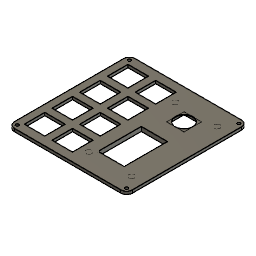
Top Plate (Autodesk Fusion 360 design; units mm, degrees)
part number: 2026-05-17-10-10-12-602
Autodesk Fusion 360 part; units mm, degrees
(part 1 of 3)
box "BoxPrimitive1" add length 100 width 50 height 2.5 placed x (0, 0, 1) y (1, 0, 0) z (0, 1, 0) at (0, 0, 0)
sketch "Sketch2" plane through (0, 2.5, 0) normal (0, 1, 0) x (-1, 0, 0)
  line L0 (0, 100) -> (-50, 100)
  line L1 (-50, 100) -> (-50, 0)
  line L2 (-50, 0) -> (0, 0)
  line L3 (0, 0) -> (0, 100)
  line L4 (-5, 95) -> (-19, 95)
  line L5 (-19, 95) -> (-19, 81)
  line L6 (-19, 81) -> (-5, 81)
  line L7 (-5, 81) -> (-5, 95)
  line L8 (-5, 95) -> (-19, 81) construction
  line L9 (-19, 95) -> (-5, 81) construction
  line L10 (-24.05, 95) -> (-38.05, 95)
  line L11 (-38.05, 95) -> (-38.05, 81)
  line L12 (-38.05, 81) -> (-24.05, 81)
  line L13 (-24.05, 81) -> (-24.05, 95)
  line L14 (-24.05, 95) -> (-38.05, 81) construction
  line L15 (-38.05, 95) -> (-24.05, 81) construction
  line L16 (-12, 88) -> (-31.05, 88)
  line L17 (-31.05, 88) -> (-31.05, 68.95)
  line L18 (-24.05, 75.95) -> (-38.05, 75.95)
  line L19 (-38.05, 75.95) -> (-38.05, 61.95)
  line L20 (-38.05, 61.95) -> (-24.05, 61.95)
  line L21 (-24.05, 61.95) -> (-24.05, 75.95)
  line L22 (-24.05, 75.95) -> (-38.05, 61.95) construction
  line L23 (-38.05, 75.95) -> (-24.05, 61.95) construction
  line L24 (-31.05, 68.95) -> (-31.05, 49.9)
  line L25 (-31.05, 49.9) -> (-12, 49.9)
  line L26 (-12, 49.9) -> (-12, 30.85)
  line L27 (-12, 30.85) -> (-31.05, 30.85)
  line L28 (-31.05, 30.85) -> (-31.05, 11.8)
  line L29 (-31.05, 11.8) -> (-12, 11.8)
  line L30 (-12, 49.9) -> (-12, 68.95)
  line L31 (-5, 61.95) -> (-19, 61.95)
  line L32 (-19, 61.95) -> (-19, 75.95)
  line L33 (-19, 75.95) -> (-5, 75.95)
  line L34 (-5, 75.95) -> (-5, 61.95)
  line L35 (-5, 61.95) -> (-19, 75.95) construction
  line L36 (-19, 61.95) -> (-5, 75.95) construction
  line L37 (-5, 56.9) -> (-19, 56.9)
  line L38 (-19, 56.9) -> (-19, 42.9)
  line L39 (-19, 42.9) -> (-5, 42.9)
  line L40 (-5, 42.9) -> (-5, 56.9)
  line L41 (-5, 56.9) -> (-19, 42.9) construction
  line L42 (-19, 56.9) -> (-5, 42.9) construction
  line L43 (-24.05, 42.9) -> (-38.05, 42.9)
  line L44 (-38.05, 42.9) -> (-38.05, 56.9)
  line L45 (-38.05, 56.9) -> (-24.05, 56.9)
  line L46 (-24.05, 56.9) -> (-24.05, 42.9)
  line L47 (-24.05, 42.9) -> (-38.05, 56.9) construction
  line L48 (-38.05, 42.9) -> (-24.05, 56.9) construction
  line L49 (-24.05, 23.85) -> (-38.05, 23.85)
  line L50 (-38.05, 23.85) -> (-38.05, 37.85)
  line L51 (-38.05, 37.85) -> (-24.05, 37.85)
  line L52 (-24.05, 37.85) -> (-24.05, 23.85)
  line L53 (-24.05, 23.85) -> (-38.05, 37.85) construction
  line L54 (-38.05, 23.85) -> (-24.05, 37.85) construction
  line L55 (-5, 23.85) -> (-19, 23.85)
  line L56 (-19, 23.85) -> (-19, 37.85)
  line L57 (-19, 37.85) -> (-5, 37.85)
  line L58 (-5, 37.85) -> (-5, 23.85)
  line L59 (-5, 23.85) -> (-19, 37.85) construction
  line L60 (-19, 23.85) -> (-5, 37.85) construction
  point P0 (-12, 88)
  point P1 (-31.05, 88)
  point P2 (-31.05, 68.95)
  point P3 (-12, 68.95)
  point P4 (-12, 49.9)
  point P5 (-31.05, 49.9)
  point P6 (-31.05, 30.85)
  point P7 (-12, 30.85)
  dimension "d8" = 14
  dimension "d9" = 14
  dimension "d10" = 14
  dimension "d11" = 14
  dimension "d12" = 19.05
  dimension "d13" = 19.05
  dimension "d14" = 14
  dimension "d15" = 14
  dimension "d16" = 19.05
  dimension "d17" = 19.05
  dimension "d18" = 19.05
  dimension "d19" = 19.05
  dimension "d20" = 19.05
  dimension "d21" = 19.05
  dimension "d22" = 19.05
  dimension "d23" = 14
  dimension "d24" = 14
  dimension "d25" = 14
  dimension "d26" = 14
  dimension "d27" = 14
  dimension "d28" = 14
  dimension "d29" = 14
  dimension "d30" = 14
  dimension "d31" = 14
  dimension "d32" = 14
  constraint horizontal L4
  constraint perpendicular L4 L5
  constraint parallel L4 L6
  constraint parallel L5 L7
  constraint coincident L8 P0
  constraint coincident L9 P0
  constraint horizontal L10
  constraint perpendicular L10 L11
  constraint parallel L10 L12
  constraint parallel L11 L13
  constraint coincident L14 P1
  constraint coincident L15 P1
  constraint coincident P0 L16.start
  constraint parallel L6 L16
  constraint coincident P1 L16.end
  constraint perpendicular L12 L17
  constraint horizontal L18
  constraint perpendicular L18 L19
  constraint parallel L18 L20
  constraint parallel L19 L21
  constraint coincident L22 P2
  constraint coincident L23 P2
  constraint coincident P2 L17.end
  constraint perpendicular L20 L24
  constraint perpendicular L24 L25
  constraint perpendicular L25 L26
  constraint perpendicular L26 L27
  constraint perpendicular L27 L28
  constraint perpendicular L28 L29
  constraint perpendicular L25 L30
  constraint horizontal L31
  constraint perpendicular L31 L32
  constraint parallel L31 L33
  constraint parallel L32 L34
  constraint coincident L35 P3
  constraint coincident L36 P3
  constraint coincident P3 L30.end
  constraint horizontal L37
  constraint perpendicular L37 L38
  constraint parallel L37 L39
  constraint parallel L38 L40
  constraint coincident L41 P4
  constraint coincident L42 P4
  constraint coincident P4 L25.end
  constraint horizontal L43
  constraint perpendicular L43 L44
  constraint parallel L43 L45
  constraint parallel L44 L46
  constraint coincident L47 P5
  constraint coincident L48 P5
  constraint coincident P5 L24.end
  constraint horizontal L49
  constraint perpendicular L49 L50
  constraint parallel L49 L51
  constraint parallel L50 L52
  constraint coincident L53 P6
  constraint coincident L54 P6
  constraint coincident P6 L27.end
  constraint horizontal L55
  constraint perpendicular L55 L56
  constraint parallel L55 L57
  constraint parallel L56 L58
  constraint coincident L59 P7
  constraint coincident L60 P7
  constraint coincident P7 L26.end
  measures "d8" distance of L5.end L6.end
  measures "d9" distance of L4.end L5.end
  measures "d10" distance of L11.end L12.end
  measures "d11" distance of L10.end L11.end
  measures "d12" distance of P0 P1
  measures "d13" distance of P1 P2
  measures "d14" distance of L19.end L20.end
  measures "d15" distance of L18.end L19.end
  measures "d16" distance of P2 P5
  measures "d17" distance of P5 P4
  measures "d18" distance of P4 P7
  measures "d19" distance of P7 P6
  measures "d20" distance of P6 L28.end
  measures "d21" distance of L28.end L29.end
  measures "d22" distance of P4 P3
  measures "d23" distance of L32.end L33.end
  measures "d24" distance of L31.end L32.end
  measures "d25" distance of L38.end L39.end
  measures "d26" distance of L37.end L38.end
  measures "d27" distance of L44.end L45.end
  measures "d28" distance of L43.end L44.end
  measures "d29" distance of L50.end L51.end
  measures "d30" distance of L49.end L50.end
  measures "d31" distance of L56.end L57.end
  measures "d32" distance of L55.end L56.end
extrude "Extrude1" cut sketch "Sketch2" against normal blind 10 contours L4 L5 L6 L7 | L10 L11 L12 L13 L16 L17 | L12 L13 L16 L17 | L17 L18 L20 L21 L24 | L17 L18 L19 L20 L24 | L24 L25 L45 L46 | L24 L25 L43 L44 L45 L46 | L25 L30 L37 L38 | L25 L26 L38 L39 | L26 L30 L37 L39 L40 | L26 L27 L55 L56 L57 L58 | L26 L27 L56 L57 | L27 L28 L49 L52 | L27 L28 L49 L50 L51 L52 | L31 L32 L33 L34
sketch "Sketch3" plane through (0, 2.5, 0) normal (0, 1, 0) x (-1, 0, 0)
  line L0 (0, 100) -> (-50, 100)
  line L1 (-50, 100) -> (-50, 0)
  line L2 (-50, 0) -> (0, 0)
  line L3 (0, 0) -> (0, 100)
  line L4 (-38.05, 95) -> (-24.05, 95)
  line L5 (-24.05, 95) -> (-24.05, 81)
  line L6 (-24.05, 81) -> (-38.05, 81)
  line L7 (-38.05, 81) -> (-38.05, 95)
  line L8 (-19, 61.95) -> (-19, 75.95)
  line L9 (-19, 75.95) -> (-5, 75.95)
  line L10 (-5, 75.95) -> (-5, 61.95)
  line L11 (-5, 61.95) -> (-19, 61.95)
  line L12 (-38.05, 23.85) -> (-38.05, 37.85)
  line L13 (-38.05, 37.85) -> (-24.05, 37.85)
  line L14 (-24.05, 37.85) -> (-24.05, 23.85)
  line L15 (-24.05, 23.85) -> (-38.05, 23.85)
  line L16 (-19, 95) -> (-5, 95)
  line L17 (-5, 95) -> (-5, 81)
  line L18 (-5, 81) -> (-19, 81)
  line L19 (-19, 81) -> (-19, 95)
  line L20 (-38.05, 75.95) -> (-24.05, 75.95)
  line L21 (-24.05, 75.95) -> (-24.05, 61.95)
  line L22 (-24.05, 61.95) -> (-38.05, 61.95)
  line L23 (-38.05, 61.95) -> (-38.05, 75.95)
  line L24 (-19, 56.9) -> (-5, 56.9)
  line L25 (-5, 56.9) -> (-5, 42.9)
  line L26 (-5, 42.9) -> (-19, 42.9)
  line L27 (-19, 42.9) -> (-19, 56.9)
  line L28 (-19, 23.85) -> (-19, 37.85)
  line L29 (-19, 37.85) -> (-5, 37.85)
  line L30 (-5, 37.85) -> (-5, 23.85)
  line L31 (-5, 23.85) -> (-19, 23.85)
  line L32 (-38.05, 42.9) -> (-38.05, 56.9)
  line L33 (-38.05, 56.9) -> (-24.05, 56.9)
  line L34 (-24.05, 56.9) -> (-24.05, 42.9)
  line L35 (-24.05, 42.9) -> (-38.05, 42.9)
  line L36 (-38.05, 23.85) -> (-38.05, 18.85)
  line L37 (-38.05, 18.85) -> (-43.05, 18.85)
  line L38 (-43.05, 18.85) -> (0, 18.85)
  line L39 (0, 18.85) -> (0, 100)
  line L40 (0, 100) -> (-43.05, 100)
  line L41 (-43.05, 100) -> (-43.05, 18.85)
  dimension "d35" = 5
  dimension "d36" = 5
  constraint coincident L12.start L15.end
  constraint perpendicular L15 L36
  constraint perpendicular L36 L37
  constraint horizontal L38
  constraint vertical L39
  constraint horizontal L40
  constraint vertical L41
  constraint coincident L0.start L3.end
  measures "d35" distance of L12.start L36.end
  measures "d36" distance of L36.end L37.end
extrude "Extrude2" cut sketch "Sketch3" against normal blind 10 contours L0 L1 L2 L3 L37 L38 L41
extrude "Extrude3" add 1 faces at (43.05, 1.6667, 72.95) along direction (1, 0, 0) blind 35.03
extrude "Extrude4" add 1 faces at (78.08, 1.6667, 72.95) along direction (1, 0, 0) blind 5
sketch "Sketch4" plane through (0, 2.5, 0) normal (0, 1, 0) x (-1, 0, 0)
  line L0 (-83.08, 18.85) -> (0, 18.85)
  line L1 (0, 18.85) -> (0, 100)
  line L2 (0, 100) -> (-83.08, 100)
  line L3 (-83.08, 100) -> (-83.08, 18.85)
  line L4 (-38.05, 42.9) -> (-38.05, 56.9)
  line L5 (-38.05, 56.9) -> (-24.05, 56.9)
  line L6 (-24.05, 56.9) -> (-24.05, 42.9)
  line L7 (-24.05, 42.9) -> (-38.05, 42.9)
  line L8 (-19, 23.85) -> (-19, 37.85)
  line L9 (-19, 37.85) -> (-5, 37.85)
  line L10 (-5, 37.85) -> (-5, 23.85)
  line L11 (-5, 23.85) -> (-19, 23.85)
  line L12 (-19, 56.9) -> (-5, 56.9)
  line L13 (-5, 56.9) -> (-5, 42.9)
  line L14 (-5, 42.9) -> (-19, 42.9)
  line L15 (-19, 42.9) -> (-19, 56.9)
  line L16 (-38.05, 75.95) -> (-24.05, 75.95)
  line L17 (-24.05, 75.95) -> (-24.05, 61.95)
  line L18 (-24.05, 61.95) -> (-38.05, 61.95)
  line L19 (-38.05, 61.95) -> (-38.05, 75.95)
  line L20 (-19, 95) -> (-5, 95)
  line L21 (-5, 95) -> (-5, 81)
  line L22 (-5, 81) -> (-19, 81)
  line L23 (-19, 81) -> (-19, 95)
  line L24 (-38.05, 23.85) -> (-38.05, 37.85)
  line L25 (-38.05, 37.85) -> (-24.05, 37.85)
  line L26 (-24.05, 37.85) -> (-24.05, 23.85)
  line L27 (-24.05, 23.85) -> (-38.05, 23.85)
  line L28 (-19, 61.95) -> (-19, 75.95)
  line L29 (-19, 75.95) -> (-5, 75.95)
  line L30 (-5, 75.95) -> (-5, 61.95)
  line L31 (-5, 61.95) -> (-19, 61.95)
  line L32 (-38.05, 95) -> (-24.05, 95)
  line L33 (-24.05, 95) -> (-24.05, 81)
  line L34 (-24.05, 81) -> (-38.05, 81)
  line L35 (-38.05, 81) -> (-38.05, 95)
  line L36 (-83.08, 18.85) -> (-83.08, 26.975)
  line L37 (-38, 100) -> (-38, 91.875)
  line L38 (-83.08, 26.975) -> (-78.08, 26.975)
  line L39 (-38, 91.875) -> (-43, 91.875)
  line L40 (-43, 91.875) -> (-78.08, 91.875)
  line L41 (-78.08, 91.875) -> (-78.08, 26.975)
  line L42 (-78.08, 26.975) -> (-43, 26.975)
  line L43 (-43, 26.975) -> (-43, 91.875)
  line L44 (-43, 91.875) -> (-43, 87.865)
  line L45 (-43, 87.865) -> (-49.05, 87.865)
  line L46 (-49.05, 87.865) -> (-49.05, 52.815)
  line L47 (-49.05, 87.865) -> (-52.98, 87.865)
  line L48 (-52.98, 87.865) -> (-52.98, 83.865)
  line L49 (-52.98, 83.865) -> (-71.9, 83.865)
  line L50 (-71.9, 83.865) -> (-71.9, 56.225)
  line L51 (-71.9, 56.225) -> (-52.98, 56.225)
  line L52 (-52.98, 56.225) -> (-52.98, 83.865)
  dimension "d43" = 8.125
  dimension "d44" = 8.125
  dimension "d45" = 5
  dimension "d46" = 5
  dimension "d47" = 4.01
  dimension "d48" = 6.05
  dimension "d49" = 35.05
  dimension "d50" = 3.93
  dimension "d51" = 4
  dimension "d52" = 18.92
  dimension "d53" = 27.64
  constraint coincident L0.start L3.end
  constraint perpendicular L0 L36
  constraint coincident L2 L37.start
  constraint perpendicular L2 L37
  constraint perpendicular L3 L38
  constraint perpendicular L35 L39
  constraint horizontal L40
  constraint vertical L41
  constraint horizontal L42
  constraint vertical L43
  constraint perpendicular L40 L44
  constraint perpendicular L44 L45
  constraint perpendicular L45 L46
  constraint perpendicular L46 L47
  constraint perpendicular L45 L48
  constraint horizontal L49
  constraint vertical L50
  constraint horizontal L51
  constraint vertical L52
  measures "d43" distance of L0.start L36.end
  measures "d44" distance of L37.start L37.end
  measures "d45" distance of L36.end L38.end
  measures "d46" distance of L37.end L39.end
  measures "d47" distance of L39.end L44.end
  measures "d48" distance of L44.end L45.end
  measures "d49" distance of L45.end L46.end
  measures "d50" distance of L45.end L47.end
  measures "d51" distance of L47.end L48.end
  measures "d52" distance of L48.end L49.end
  measures "d53" distance of L48.end L51.end
extrude "Extrude5" cut sketch "Sketch4" against normal blind 6 contours L49 L50 L51 L52
sketch "Sketch5" plane through (0, 2.5, 0) normal (0, 1, 0) x (-1, 0, 0)
  line L0 (-38.05, 95) -> (-24.05, 95)
  line L1 (-24.05, 95) -> (-24.05, 81)
  line L2 (-24.05, 81) -> (-38.05, 81)
  line L3 (-38.05, 81) -> (-38.05, 95)
  line L4 (-19, 61.95) -> (-19, 75.95)
  line L5 (-19, 75.95) -> (-5, 75.95)
  line L6 (-5, 75.95) -> (-5, 61.95)
  line L7 (-5, 61.95) -> (-19, 61.95)
  line L8 (-38.05, 23.85) -> (-38.05, 37.85)
  line L9 (-38.05, 37.85) -> (-24.05, 37.85)
  line L10 (-24.05, 37.85) -> (-24.05, 23.85)
  line L11 (-24.05, 23.85) -> (-38.05, 23.85)
  line L12 (-19, 95) -> (-5, 95)
  line L13 (-5, 95) -> (-5, 81)
  line L14 (-5, 81) -> (-19, 81)
  line L15 (-19, 81) -> (-19, 95)
  line L16 (-38.05, 75.95) -> (-24.05, 75.95)
  line L17 (-24.05, 75.95) -> (-24.05, 61.95)
  line L18 (-24.05, 61.95) -> (-38.05, 61.95)
  line L19 (-38.05, 61.95) -> (-38.05, 75.95)
  line L20 (-19, 56.9) -> (-5, 56.9)
  line L21 (-5, 56.9) -> (-5, 42.9)
  line L22 (-5, 42.9) -> (-19, 42.9)
  line L23 (-19, 42.9) -> (-19, 56.9)
  line L24 (-19, 23.85) -> (-19, 37.85)
  line L25 (-19, 37.85) -> (-5, 37.85)
  line L26 (-5, 37.85) -> (-5, 23.85)
  line L27 (-5, 23.85) -> (-19, 23.85)
  line L28 (-38.05, 42.9) -> (-38.05, 56.9)
  line L29 (-38.05, 56.9) -> (-24.05, 56.9)
  line L30 (-24.05, 56.9) -> (-24.05, 42.9)
  line L31 (-24.05, 42.9) -> (-38.05, 42.9)
  line L32 (-83.08, 18.85) -> (0, 18.85)
  line L33 (0, 18.85) -> (0, 100)
  line L34 (0, 100) -> (-83.08, 100)
  line L35 (-83.08, 100) -> (-83.08, 18.85)
  line L36 (-71.9, 83.865) -> (-52.98, 83.865)
  line L37 (-52.98, 83.865) -> (-52.98, 56.225)
  line L38 (-52.98, 56.225) -> (-71.9, 56.225)
  line L39 (-71.9, 56.225) -> (-71.9, 83.865)
  line L40 (-78.067, 18.85) -> (-78.067, 26.975)
  line L41 (-78.067, 26.975) -> (-83.067, 26.975)
  line L42 (-43.0945, 100) -> (-43.0945, 91.875)
  line L43 (-43.0945, 91.875) -> (-38.0945, 91.875)
  line L44 (-43.0945, 91.875) -> (-78.067, 91.875)
  line L45 (-78.067, 91.875) -> (-78.067, 26.975)
  line L46 (-78.067, 26.975) -> (-43.0945, 26.975)
  line L47 (-43.0945, 26.975) -> (-43.0945, 91.875)
  line L48 (-43.0945, 26.975) -> (-43.0945, 41.635)
  line L49 (-78.067, 26.975) -> (-78.067, 41.635)
  line L50 (-78.067, 41.635) -> (-74.177, 41.635)
  line L51 (-43.0945, 41.635) -> (-46.9845, 41.635)
  line L52 (-46.9845, 41.635) -> (-50.6145, 41.635)
  line L53 (-50.6145, 41.635) -> (-50.6145, 35.535)
  line L54 (-50.6145, 35.535) -> (-46.9845, 35.535)
  line L55 (-46.9845, 35.535) -> (-46.9845, 41.635)
  line L56 (-74.177, 41.635) -> (-70.547, 41.635)
  line L57 (-70.547, 41.635) -> (-70.547, 35.535)
  line L58 (-70.547, 35.535) -> (-74.177, 35.535)
  line L59 (-74.177, 35.535) -> (-74.177, 41.635)
  line L60 (-60.7555, 26.975) -> (-60.7555, 38.585)
  line L61 (-60.7555, 38.585) -> (-43.1555, 38.585)
  circle A0 centre (-60.7555, 38.585) radius 3.5
  line L62 (-64.2555, 42.085) -> (-57.2555, 42.085)
  line L63 (-57.2555, 42.085) -> (-57.2555, 35.085)
  line L64 (-57.2555, 35.085) -> (-64.2555, 35.085)
  line L65 (-64.2555, 35.085) -> (-64.2555, 42.085)
  line L66 (-64.2555, 42.085) -> (-57.2555, 35.085) construction
  line L67 (-57.2555, 42.085) -> (-64.2555, 35.085) construction
  point P0 (-60.7555, 38.585)
  dimension "d58" = 8.125
  dimension "d59" = 5
  dimension "d60" = 8.125
  dimension "d61" = 5
  dimension "d62" = 14.66
  dimension "d63" = 14.66
  dimension "d64" = 3.89
  dimension "d65" = 3.89
  dimension "d66" = 3.63
  dimension "d67" = 6.1
  dimension "d68" = 3.63
  dimension "d69" = 6.1
  dimension "d70" = 11.61
  dimension "d71" = 17.6
  dimension "d72" = 7
  dimension "d73" = 7
  dimension "d74" = 7
  constraint coincident L32 L40.start
  constraint perpendicular L32 L40
  constraint perpendicular L40 L41
  constraint coincident L34 L42.start
  constraint perpendicular L34 L42
  constraint perpendicular L42 L43
  constraint horizontal L44
  constraint vertical L45
  constraint horizontal L46
  constraint vertical L47
  constraint perpendicular L46 L48
  constraint perpendicular L46 L49
  constraint perpendicular L45 L50
  constraint perpendicular L47 L51
  constraint horizontal L52
  constraint vertical L53
  constraint horizontal L54
  constraint vertical L55
  constraint horizontal L56
  constraint vertical L57
  constraint horizontal L58
  constraint vertical L59
  constraint coincident L46 L60.start
  constraint perpendicular L46 L60
  constraint perpendicular L60 L61
  constraint coincident P0 L60.end
  constraint horizontal L62
  constraint perpendicular L62 L63
  constraint parallel L62 L64
  constraint parallel L63 L65
  constraint coincident L66 P0
  constraint coincident L67 P0
  measures "d58" distance of L40.start L40.end
  measures "d59" distance of L40.end L41.end
  measures "d60" distance of L42.start L42.end
  measures "d61" distance of L42.end L43.end
  measures "d62" distance of L46.end L48.end
  measures "d63" distance of L40.end L49.end
  measures "d64" distance of L49.end L50.end
  measures "d65" distance of L48.end L51.end
  measures "d66" distance of L51.end L52.end
  measures "d67" distance of L51.end L54.end
  measures "d68" distance of L50.end L56.end
  measures "d69" distance of L50.end L58.end
  measures "d70" distance of L60.start P0
  measures "d71" distance of P0 L61.end
  measures "d72" diameter of A0
  measures "d73" distance of L63.end L64.end
  measures "d74" distance of L62.end L63.end
extrude "Extrude6" cut sketch "Sketch5" against normal blind 6 contours L60 L61 A0 | A0 L64 L65 | L60 L61 A0 | A0 L63 L64 | A0 L62 L65 | A0 L62 L63 | L52 L53 L55 L61 | L53 L54 L55 L61 | L56 L57 L58 L59
extrude "Extrude7" cut 1 faces at (59.4618, 2.5, 25.9283) along direction (0, -1, 0) blind 0.5
sketch "Sketch6" plane through (0, 0, 0) normal (0, -1, 0) x (1, 0, 0)
  line L0 (52.98, 83.865) -> (71.9, 83.865)
  line L1 (71.9, 83.865) -> (71.9, 56.225)
  line L2 (71.9, 56.225) -> (52.98, 56.225)
  line L3 (52.98, 56.225) -> (52.98, 83.865)
  line L4 (38.05, 56.9) -> (38.05, 42.9)
  line L5 (38.05, 42.9) -> (24.05, 42.9)
  line L6 (24.05, 42.9) -> (24.05, 56.9)
  line L7 (24.05, 56.9) -> (38.05, 56.9)
  line L8 (19, 37.85) -> (19, 23.85)
  line L9 (19, 23.85) -> (5, 23.85)
  line L10 (5, 23.85) -> (5, 37.85)
  line L11 (5, 37.85) -> (19, 37.85)
  line L12 (5, 56.9) -> (19, 56.9)
  line L13 (19, 56.9) -> (19, 42.9)
  line L14 (19, 42.9) -> (5, 42.9)
  line L15 (5, 42.9) -> (5, 56.9)
  line L16 (24.05, 75.95) -> (38.05, 75.95)
  line L17 (38.05, 75.95) -> (38.05, 61.95)
  line L18 (38.05, 61.95) -> (24.05, 61.95)
  line L19 (24.05, 61.95) -> (24.05, 75.95)
  line L20 (5, 95) -> (19, 95)
  line L21 (19, 95) -> (19, 81)
  line L22 (19, 81) -> (5, 81)
  line L23 (5, 81) -> (5, 95)
  line L24 (38.05, 37.85) -> (38.05, 23.85)
  line L25 (38.05, 23.85) -> (24.05, 23.85)
  line L26 (24.05, 23.85) -> (24.05, 37.85)
  line L27 (24.05, 37.85) -> (38.05, 37.85)
  line L28 (19, 75.95) -> (19, 61.95)
  line L29 (19, 61.95) -> (5, 61.95)
  line L30 (5, 61.95) -> (5, 75.95)
  line L31 (5, 75.95) -> (19, 75.95)
  line L32 (24.05, 95) -> (38.05, 95)
  line L33 (38.05, 95) -> (38.05, 81)
  line L34 (38.05, 81) -> (24.05, 81)
  line L35 (24.05, 81) -> (24.05, 95)
  line L36 (83.08, 100) -> (0, 100)
  line L37 (0, 100) -> (0, 18.85)
  line L38 (0, 18.85) -> (83.08, 18.85)
  line L39 (83.08, 18.85) -> (83.08, 100)
  line L40 (70.547, 35.535) -> (70.547, 41.635)
  line L41 (70.547, 41.635) -> (74.177, 41.635)
  line L42 (74.177, 41.635) -> (74.177, 35.535)
  line L43 (74.177, 35.535) -> (70.547, 35.535)
  line L44 (57.2555, 35.085) -> (57.2555, 42.085)
  line L45 (57.2555, 42.085) -> (64.2555, 42.085)
  line L46 (64.2555, 42.085) -> (64.2555, 35.085)
  line L47 (64.2555, 35.085) -> (57.2555, 35.085)
  line L48 (46.9845, 41.635) -> (50.6145, 41.635)
  line L49 (50.6145, 41.635) -> (50.6145, 35.535)
  line L50 (50.6145, 35.535) -> (46.9845, 35.535)
  line L51 (46.9845, 35.535) -> (46.9845, 41.635)
  line L52 (43.0348, 18.85) -> (43.0348, 26.975)
  line L53 (43.0348, 26.975) -> (38.0348, 26.975)
  line L54 (78.0935, 100) -> (78.0935, 91.875)
  line L55 (78.0935, 91.875) -> (83.0935, 91.875)
  line L56 (78.0935, 91.875) -> (43.0348, 91.875)
  line L57 (43.0348, 91.875) -> (43.0348, 26.975)
  line L58 (43.0348, 26.975) -> (78.0935, 26.975)
  line L59 (78.0935, 26.975) -> (78.0935, 91.875)
  line L60 (75.1296, 91.875) -> (75.1296, 88.925)
  line L61 (75.1296, 88.925) -> (78.0996, 88.925)
  line L62 (43.0348, 91.875) -> (43.0348, 89.005)
  line L63 (43.0348, 89.005) -> (45.8848, 89.005)
  line L64 (78.0935, 26.975) -> (78.0935, 29.945)
  line L65 (78.0935, 29.945) -> (74.9435, 29.945)
  line L66 (43.0348, 26.975) -> (43.0348, 29.975)
  line L67 (43.0348, 29.975) -> (45.9348, 29.975)
  circle A0 centre (45.9348, 29.975) radius 1.85
  circle A1 centre (74.9435, 29.945) radius 1.85
  circle A2 centre (75.1296, 88.925) radius 1.85
  circle A3 centre (45.8848, 89.005) radius 1.85
  dimension "d79" = 8.125
  dimension "d80" = 5
  dimension "d81" = 8.125
  dimension "d82" = 5
  dimension "d85" = 2.95
  dimension "d86" = 2.97
  dimension "d87" = 2.87
  dimension "d88" = 2.85
  dimension "d89" = 2.97
  dimension "d90" = 3.15
  dimension "d91" = 3
  dimension "d92" = 2.9
  dimension "d93" = 3.7
  dimension "d94" = 3.7
  dimension "d95" = 3.7
  dimension "d96" = 3.7
  constraint coincident L38 L52.start
  constraint perpendicular L38 L52
  constraint perpendicular L52 L53
  constraint coincident L36 L54.start
  constraint perpendicular L36 L54
  constraint perpendicular L54 L55
  constraint horizontal L56
  constraint vertical L57
  constraint horizontal L58
  constraint vertical L59
  constraint coincident L56 L60.start
  constraint perpendicular L56 L60
  constraint perpendicular L59 L61
  constraint perpendicular L56 L62
  constraint perpendicular L62 L63
  constraint perpendicular L58 L64
  constraint perpendicular L64 L65
  constraint perpendicular L58 L66
  constraint perpendicular L66 L67
  constraint coincident L67.end A0.centre
  constraint coincident L65.end A1.centre
  constraint coincident L60.end L61.start
  constraint coincident L63.end A3.centre
  measures "d79" distance of L52.start L52.end
  measures "d80" distance of L52.end L53.end
  measures "d81" distance of L54.start L54.end
  measures "d82" distance of L54.end L55.end
  measures "d85" distance of L60.start L60.end
  measures "d86" distance of L60.end L61.end
  measures "d87" distance of L56.end L62.end
  measures "d88" distance of L62.end L63.end
  measures "d89" distance of L58.end L64.end
  measures "d90" distance of L64.end L65.end
  measures "d91" distance of L52.end L66.end
  measures "d92" distance of L66.end L67.end
  measures "d93" diameter of A0
  measures "d94" diameter of A1
  measures "d95" diameter of A2
  measures "d96" diameter of A3
extrude "Extrude8" add 1 faces at (59.4618, 2, 25.9283) along direction (0, 1, 0) blind 1
extrude "Extrude9" cut sketch "Sketch6" against normal blind 4 contours L60 L61 A2 | L60 L61 A2 | A0 | A1 | A3
sketch "Sketch7" plane through (0, 3, 0) normal (0, 1, 0) x (-1, 0, 0)
  line L0 (-50.6145, 41.635) -> (-46.9845, 41.635)
  line L1 (-46.9845, 41.635) -> (-46.9845, 35.535)
  line L2 (-46.9845, 35.535) -> (-50.6145, 35.535)
  line L3 (-50.6145, 35.535) -> (-50.6145, 41.635)
  line L4 (-57.2555, 42.085) -> (-57.2555, 35.085)
  line L5 (-57.2555, 35.085) -> (-64.2555, 35.085)
  line L6 (-64.2555, 35.085) -> (-64.2555, 42.085)
  line L7 (-64.2555, 42.085) -> (-57.2555, 42.085)
  line L8 (-70.547, 41.635) -> (-70.547, 35.535)
  line L9 (-70.547, 35.535) -> (-74.177, 35.535)
  line L10 (-74.177, 35.535) -> (-74.177, 41.635)
  line L11 (-74.177, 41.635) -> (-70.547, 41.635)
  line L12 (-38.05, 95) -> (-24.05, 95)
  line L13 (-24.05, 95) -> (-24.05, 81)
  line L14 (-24.05, 81) -> (-38.05, 81)
  line L15 (-38.05, 81) -> (-38.05, 95)
  line L16 (-19, 61.95) -> (-19, 75.95)
  line L17 (-19, 75.95) -> (-5, 75.95)
  line L18 (-5, 75.95) -> (-5, 61.95)
  line L19 (-5, 61.95) -> (-19, 61.95)
  line L20 (-38.05, 23.85) -> (-38.05, 37.85)
  line L21 (-38.05, 37.85) -> (-24.05, 37.85)
  line L22 (-24.05, 37.85) -> (-24.05, 23.85)
  line L23 (-24.05, 23.85) -> (-38.05, 23.85)
  line L24 (-19, 95) -> (-5, 95)
  line L25 (-5, 95) -> (-5, 81)
  line L26 (-5, 81) -> (-19, 81)
  line L27 (-19, 81) -> (-19, 95)
  line L28 (-38.05, 75.95) -> (-24.05, 75.95)
  line L29 (-24.05, 75.95) -> (-24.05, 61.95)
  line L30 (-24.05, 61.95) -> (-38.05, 61.95)
  line L31 (-38.05, 61.95) -> (-38.05, 75.95)
  line L32 (-19, 56.9) -> (-5, 56.9)
  line L33 (-5, 56.9) -> (-5, 42.9)
  line L34 (-5, 42.9) -> (-19, 42.9)
  line L35 (-19, 42.9) -> (-19, 56.9)
  line L36 (-19, 23.85) -> (-19, 37.85)
  line L37 (-19, 37.85) -> (-5, 37.85)
  line L38 (-5, 37.85) -> (-5, 23.85)
  line L39 (-5, 23.85) -> (-19, 23.85)
  line L40 (-38.05, 42.9) -> (-38.05, 56.9)
  line L41 (-38.05, 56.9) -> (-24.05, 56.9)
  line L42 (-24.05, 56.9) -> (-24.05, 42.9)
  line L43 (-24.05, 42.9) -> (-38.05, 42.9)
  line L44 (-83.08, 18.85) -> (0, 18.85)
  line L45 (0, 18.85) -> (0, 100)
  line L46 (0, 100) -> (-83.08, 100)
  line L47 (-83.08, 100) -> (-83.08, 18.85)
  line L48 (-71.9, 83.865) -> (-52.98, 83.865)
  line L49 (-52.98, 83.865) -> (-52.98, 56.225)
  line L50 (-52.98, 56.225) -> (-71.9, 56.225)
  line L51 (-71.9, 56.225) -> (-71.9, 83.865)
  circle A0 centre (-74.9435, 29.945) radius 1.85
  circle A1 centre (-75.1296, 88.925) radius 1.85
  circle A2 centre (-45.9348, 29.975) radius 1.85
  circle A3 centre (-45.8848, 89.005) radius 1.85
  line L52 (-2.9679, 18.85) -> (-2.9679, 21.85)
  line L53 (-2.9679, 21.85) -> (0.0321, 21.85)
  circle A4 centre (-2.9679, 21.85) radius 1.5
  line L54 (-80.08, 18.85) -> (-80.08, 21.85)
  line L55 (-80.08, 21.85) -> (-83.08, 21.85)
  circle A5 centre (-80.08, 21.85) radius 1.5
  line L56 (-83.08, 97.0008) -> (-80.08, 97.0008)
  line L57 (-80.08, 97.0008) -> (-80.08, 100.0008)
  circle A6 centre (-80.08, 97.0008) radius 1.5
  line L58 (-2.9851, 100) -> (-2.9851, 97)
  line L59 (-2.9851, 97) -> (0.0149, 97)
  circle A7 centre (-2.9851, 97) radius 1.5
  dimension "d99" = 3
  dimension "d100" = 3
  dimension "d101" = 3
  dimension "d102" = 3
  dimension "d103" = 3
  dimension "d104" = 3
  dimension "d105" = 3
  dimension "d106" = 3
  dimension "d107" = 3
  dimension "d108" = 3
  dimension "d109" = 3
  dimension "d110" = 3
  constraint coincident L44 L52.start
  constraint perpendicular L44 L52
  constraint perpendicular L52 L53
  constraint coincident L52.end L53.start
  constraint coincident L44 L54.start
  constraint perpendicular L44 L54
  constraint perpendicular L54 L55
  constraint coincident L54.end L55.start
  constraint coincident L47 L56.start
  constraint perpendicular L47 L56
  constraint perpendicular L56 L57
  constraint coincident L56.end L57.start
  constraint coincident L46 L58.start
  constraint perpendicular L46 L58
  constraint perpendicular L58 L59
  constraint coincident L58.end L59.start
  measures "d99" distance of L52.start L52.end
  measures "d100" distance of L52.end L53.end
  measures "d101" diameter of A4
  measures "d102" distance of L54.start L54.end
  measures "d103" distance of L54.end L55.end
  measures "d104" diameter of A5
  measures "d105" distance of L56.start L56.end
  measures "d106" distance of L56.end L57.end
  measures "d107" diameter of A6
  measures "d108" distance of L58.start L58.end
  measures "d109" distance of L58.end L59.end
  measures "d110" diameter of A7
extrude "Extrude10" cut sketch "Sketch7" against normal blind 5 contours L54 L55 A5 | L54 L55 A5 | L52 L53 A4 | L52 L53 A4 | L56 L57 A6 | L56 L57 A6 | L58 L59 A7 | L58 L59 A7
sketch "Sketch8" plane through (0, 0, 0) normal (0, -1, 0) x (1, 0, 0)
  circle A0 centre (45.8848, 89.005) radius 1.85
  circle A1 centre (45.9348, 29.975) radius 1.85
  circle A2 centre (75.1296, 88.925) radius 1.85
  circle A3 centre (74.9435, 29.945) radius 1.85
  line L0 (52.98, 83.865) -> (71.9, 83.865)
  line L1 (71.9, 83.865) -> (71.9, 56.225)
  line L2 (71.9, 56.225) -> (52.98, 56.225)
  line L3 (52.98, 56.225) -> (52.98, 83.865)
  line L4 (38.05, 56.9) -> (38.05, 42.9)
  line L5 (38.05, 42.9) -> (24.05, 42.9)
  line L6 (24.05, 42.9) -> (24.05, 56.9)
  line L7 (24.05, 56.9) -> (38.05, 56.9)
  line L8 (19, 37.85) -> (19, 23.85)
  line L9 (19, 23.85) -> (5, 23.85)
  line L10 (5, 23.85) -> (5, 37.85)
  line L11 (5, 37.85) -> (19, 37.85)
  line L12 (5, 56.9) -> (19, 56.9)
  line L13 (19, 56.9) -> (19, 42.9)
  line L14 (19, 42.9) -> (5, 42.9)
  line L15 (5, 42.9) -> (5, 56.9)
  line L16 (24.05, 75.95) -> (38.05, 75.95)
  line L17 (38.05, 75.95) -> (38.05, 61.95)
  line L18 (38.05, 61.95) -> (24.05, 61.95)
  line L19 (24.05, 61.95) -> (24.05, 75.95)
  line L20 (5, 95) -> (19, 95)
  line L21 (19, 95) -> (19, 81)
  line L22 (19, 81) -> (5, 81)
  line L23 (5, 81) -> (5, 95)
  line L24 (38.05, 37.85) -> (38.05, 23.85)
  line L25 (38.05, 23.85) -> (24.05, 23.85)
  line L26 (24.05, 23.85) -> (24.05, 37.85)
  line L27 (24.05, 37.85) -> (38.05, 37.85)
  line L28 (19, 75.95) -> (19, 61.95)
  line L29 (19, 61.95) -> (5, 61.95)
  line L30 (5, 61.95) -> (5, 75.95)
  line L31 (5, 75.95) -> (19, 75.95)
  line L32 (24.05, 95) -> (38.05, 95)
  line L33 (38.05, 95) -> (38.05, 81)
  line L34 (38.05, 81) -> (24.05, 81)
  line L35 (24.05, 81) -> (24.05, 95)
  line L36 (83.08, 100) -> (0, 100)
  line L37 (0, 100) -> (0, 18.85)
  line L38 (0, 18.85) -> (83.08, 18.85)
  line L39 (83.08, 18.85) -> (83.08, 100)
  line L40 (70.547, 35.535) -> (70.547, 41.635)
  line L41 (70.547, 41.635) -> (74.177, 41.635)
  line L42 (74.177, 41.635) -> (74.177, 35.535)
  line L43 (74.177, 35.535) -> (70.547, 35.535)
  line L44 (57.2555, 35.085) -> (57.2555, 42.085)
  line L45 (57.2555, 42.085) -> (64.2555, 42.085)
  line L46 (64.2555, 42.085) -> (64.2555, 35.085)
  line L47 (64.2555, 35.085) -> (57.2555, 35.085)
  line L48 (46.9845, 41.635) -> (50.6145, 41.635)
  line L49 (50.6145, 41.635) -> (50.6145, 35.535)
  line L50 (50.6145, 35.535) -> (46.9845, 35.535)
  line L51 (46.9845, 35.535) -> (46.9845, 41.635)
  circle A4 centre (80.08, 97.0008) radius 1.5
  circle A5 centre (2.9851, 97) radius 1.5
  circle A6 centre (80.08, 21.85) radius 1.5
  circle A7 centre (2.9679, 21.85) radius 1.5
  circle A8 centre (75.1296, 88.925) radius 2.5
  circle A9 centre (45.8848, 89.005) radius 2.5
  circle A10 centre (45.9348, 29.975) radius 2.5
  circle A11 centre (74.9435, 29.945) radius 2.5
  dimension "d115" = 5
  dimension "d116" = 5
  dimension "d117" = 5
  dimension "d118" = 5
  constraint concentric A2 A8
  constraint concentric A0 A9
  constraint concentric A1 A10
  constraint concentric A3 A11
  measures "d115" diameter of A8
  measures "d116" diameter of A9
  measures "d117" diameter of A10
  measures "d118" diameter of A11
sketch "Sketch9" plane through (0, 3, 0) normal (0, 1, 0) x (-1, 0, 0)
  circle A0 centre (-45.8848, 89.005) radius 1.85
  circle A1 centre (-45.9348, 29.975) radius 1.85
  circle A2 centre (-75.1296, 88.925) radius 1.85
  circle A3 centre (-74.9435, 29.945) radius 1.85
  line L0 (-71.9, 83.865) -> (-52.98, 83.865)
  line L1 (-52.98, 83.865) -> (-52.98, 56.225)
  line L2 (-52.98, 56.225) -> (-71.9, 56.225)
  line L3 (-71.9, 56.225) -> (-71.9, 83.865)
  line L4 (-83.08, 18.85) -> (0, 18.85)
  line L5 (0, 18.85) -> (0, 100)
  line L6 (0, 100) -> (-83.08, 100)
  line L7 (-83.08, 100) -> (-83.08, 18.85)
  line L8 (-38.05, 42.9) -> (-38.05, 56.9)
  line L9 (-38.05, 56.9) -> (-24.05, 56.9)
  line L10 (-24.05, 56.9) -> (-24.05, 42.9)
  line L11 (-24.05, 42.9) -> (-38.05, 42.9)
  line L12 (-19, 23.85) -> (-19, 37.85)
  line L13 (-19, 37.85) -> (-5, 37.85)
  line L14 (-5, 37.85) -> (-5, 23.85)
  line L15 (-5, 23.85) -> (-19, 23.85)
  line L16 (-19, 56.9) -> (-5, 56.9)
  line L17 (-5, 56.9) -> (-5, 42.9)
  line L18 (-5, 42.9) -> (-19, 42.9)
  line L19 (-19, 42.9) -> (-19, 56.9)
  line L20 (-38.05, 75.95) -> (-24.05, 75.95)
  line L21 (-24.05, 75.95) -> (-24.05, 61.95)
  line L22 (-24.05, 61.95) -> (-38.05, 61.95)
  line L23 (-38.05, 61.95) -> (-38.05, 75.95)
  line L24 (-19, 95) -> (-5, 95)
  line L25 (-5, 95) -> (-5, 81)
  line L26 (-5, 81) -> (-19, 81)
  line L27 (-19, 81) -> (-19, 95)
  line L28 (-38.05, 23.85) -> (-38.05, 37.85)
  line L29 (-38.05, 37.85) -> (-24.05, 37.85)
  line L30 (-24.05, 37.85) -> (-24.05, 23.85)
  line L31 (-24.05, 23.85) -> (-38.05, 23.85)
  line L32 (-19, 61.95) -> (-19, 75.95)
  line L33 (-19, 75.95) -> (-5, 75.95)
  line L34 (-5, 75.95) -> (-5, 61.95)
  line L35 (-5, 61.95) -> (-19, 61.95)
  line L36 (-38.05, 95) -> (-24.05, 95)
  line L37 (-24.05, 95) -> (-24.05, 81)
  line L38 (-24.05, 81) -> (-38.05, 81)
  line L39 (-38.05, 81) -> (-38.05, 95)
  line L40 (-70.547, 41.635) -> (-70.547, 35.535)
  line L41 (-70.547, 35.535) -> (-74.177, 35.535)
  line L42 (-74.177, 35.535) -> (-74.177, 41.635)
  line L43 (-74.177, 41.635) -> (-70.547, 41.635)
  line L44 (-57.2555, 42.085) -> (-57.2555, 35.085)
  line L45 (-57.2555, 35.085) -> (-64.2555, 35.085)
  line L46 (-64.2555, 35.085) -> (-64.2555, 42.085)
  line L47 (-64.2555, 42.085) -> (-57.2555, 42.085)
  line L48 (-50.6145, 41.635) -> (-46.9845, 41.635)
  line L49 (-46.9845, 41.635) -> (-46.9845, 35.535)
  line L50 (-46.9845, 35.535) -> (-50.6145, 35.535)
  line L51 (-50.6145, 35.535) -> (-50.6145, 41.635)
  circle A4 centre (-80.08, 97.0008) radius 1.5
  circle A5 centre (-2.9851, 97) radius 1.5
  circle A6 centre (-80.08, 21.85) radius 1.5
  circle A7 centre (-2.9679, 21.85) radius 1.5
extrude "Extrude11" add sketch "Sketch9" against normal blind 1 contours A0 | A1 | A2 | A3
extrude "Extrude12" add sketch "Sketch8" along normal blind 2 contours A8 | A9 | A10 | A11
fillet "Fillet1" radius 1 4 edges at (72.7988, 0, 89.829) (43.5539, 0, 89.909) (43.6039, 0, 30.879) (72.6127, 0, 30.849)
sketch "Sketch10" plane through (0, 3, 0) normal (0, 1, 0) x (-1, 0, 0)
  line L0 (-71.9, 83.865) -> (-52.98, 83.865)
  line L1 (-52.98, 83.865) -> (-52.98, 56.225)
  line L2 (-52.98, 56.225) -> (-71.9, 56.225)
  line L3 (-71.9, 56.225) -> (-71.9, 83.865)
  line L4 (-83.08, 18.85) -> (0, 18.85)
  line L5 (0, 18.85) -> (0, 100)
  line L6 (0, 100) -> (-83.08, 100)
  line L7 (-83.08, 100) -> (-83.08, 18.85)
  line L8 (-38.05, 42.9) -> (-38.05, 56.9)
  line L9 (-38.05, 56.9) -> (-24.05, 56.9)
  line L10 (-24.05, 56.9) -> (-24.05, 42.9)
  line L11 (-24.05, 42.9) -> (-38.05, 42.9)
  line L12 (-19, 23.85) -> (-19, 37.85)
  line L13 (-19, 37.85) -> (-5, 37.85)
  line L14 (-5, 37.85) -> (-5, 23.85)
  line L15 (-5, 23.85) -> (-19, 23.85)
  line L16 (-19, 56.9) -> (-5, 56.9)
  line L17 (-5, 56.9) -> (-5, 42.9)
  line L18 (-5, 42.9) -> (-19, 42.9)
  line L19 (-19, 42.9) -> (-19, 56.9)
  line L20 (-38.05, 75.95) -> (-24.05, 75.95)
  line L21 (-24.05, 75.95) -> (-24.05, 61.95)
  line L22 (-24.05, 61.95) -> (-38.05, 61.95)
  line L23 (-38.05, 61.95) -> (-38.05, 75.95)
  line L24 (-19, 95) -> (-5, 95)
  line L25 (-5, 95) -> (-5, 81)
  line L26 (-5, 81) -> (-19, 81)
  line L27 (-19, 81) -> (-19, 95)
  line L28 (-38.05, 23.85) -> (-38.05, 37.85)
  line L29 (-38.05, 37.85) -> (-24.05, 37.85)
  line L30 (-24.05, 37.85) -> (-24.05, 23.85)
  line L31 (-24.05, 23.85) -> (-38.05, 23.85)
  line L32 (-19, 61.95) -> (-19, 75.95)
  line L33 (-19, 75.95) -> (-5, 75.95)
  line L34 (-5, 75.95) -> (-5, 61.95)
  line L35 (-5, 61.95) -> (-19, 61.95)
  line L36 (-38.05, 95) -> (-24.05, 95)
  line L37 (-24.05, 95) -> (-24.05, 81)
  line L38 (-24.05, 81) -> (-38.05, 81)
  line L39 (-38.05, 81) -> (-38.05, 95)
  line L40 (-70.547, 41.635) -> (-70.547, 35.535)
  line L41 (-70.547, 35.535) -> (-74.177, 35.535)
  line L42 (-74.177, 35.535) -> (-74.177, 41.635)
  line L43 (-74.177, 41.635) -> (-70.547, 41.635)
  line L44 (-57.2555, 42.085) -> (-57.2555, 35.085)
  line L45 (-57.2555, 35.085) -> (-64.2555, 35.085)
  line L46 (-64.2555, 35.085) -> (-64.2555, 42.085)
  line L47 (-64.2555, 42.085) -> (-57.2555, 42.085)
  line L48 (-50.6145, 41.635) -> (-46.9845, 41.635)
  line L49 (-46.9845, 41.635) -> (-46.9845, 35.535)
  line L50 (-46.9845, 35.535) -> (-50.6145, 35.535)
  line L51 (-50.6145, 35.535) -> (-50.6145, 41.635)
  circle A0 centre (-80.08, 97.0008) radius 1.5
  circle A1 centre (-2.9851, 97) radius 1.5
  circle A2 centre (-80.08, 21.85) radius 1.5
  circle A3 centre (-2.9679, 21.85) radius 1.5
  circle A4 centre (-60.755, 38.6) radius 3.5
  dimension "d123" = 7
  measures "d123" diameter of A4
extrude "Extrude13" add sketch "Sketch10" against normal blind 3 contours L44 L47 A4 | L44 L45 L46 A4 | L46 L47 A4
sketch "Sketch11" plane through (0, 3, 0) normal (0, 1, 0) x (-1, 0, 0)
  line L0 (-71.9, 83.865) -> (-52.98, 83.865)
  line L1 (-52.98, 56.225) -> (-71.9, 56.225)
  line L2 (-71.9, 56.225) -> (-71.9, 83.865)
  line L3 (-83.08, 18.85) -> (0, 18.85)
  line L4 (0, 18.85) -> (0, 100)
  line L5 (0, 100) -> (-83.08, 100)
  line L6 (-83.08, 100) -> (-83.08, 18.85)
  line L7 (-38.05, 42.9) -> (-38.05, 56.9)
  line L8 (-38.05, 56.9) -> (-24.05, 56.9)
  line L9 (-24.05, 56.9) -> (-24.05, 42.9)
  line L10 (-24.05, 42.9) -> (-38.05, 42.9)
  line L11 (-19, 23.85) -> (-19, 37.85)
  line L12 (-19, 37.85) -> (-5, 37.85)
  line L13 (-5, 37.85) -> (-5, 23.85)
  line L14 (-5, 23.85) -> (-19, 23.85)
  line L15 (-19, 56.9) -> (-5, 56.9)
  line L16 (-5, 56.9) -> (-5, 42.9)
  line L17 (-5, 42.9) -> (-19, 42.9)
  line L18 (-19, 42.9) -> (-19, 56.9)
  line L19 (-38.05, 75.95) -> (-24.05, 75.95)
  line L20 (-24.05, 75.95) -> (-24.05, 61.95)
  line L21 (-24.05, 61.95) -> (-38.05, 61.95)
  line L22 (-38.05, 61.95) -> (-38.05, 75.95)
  line L23 (-19, 95) -> (-5, 95)
  line L24 (-5, 95) -> (-5, 81)
  line L25 (-5, 81) -> (-19, 81)
  line L26 (-19, 81) -> (-19, 95)
  line L27 (-38.05, 23.85) -> (-38.05, 37.85)
  line L28 (-38.05, 37.85) -> (-24.05, 37.85)
  line L29 (-24.05, 37.85) -> (-24.05, 23.85)
  line L30 (-24.05, 23.85) -> (-38.05, 23.85)
  line L31 (-19, 61.95) -> (-19, 75.95)
  line L32 (-19, 75.95) -> (-5, 75.95)
  line L33 (-5, 75.95) -> (-5, 61.95)
  line L34 (-5, 61.95) -> (-19, 61.95)
  line L35 (-38.05, 95) -> (-24.05, 95)
  line L36 (-24.05, 95) -> (-24.05, 81)
  line L37 (-24.05, 81) -> (-38.05, 81)
  line L38 (-38.05, 81) -> (-38.05, 95)
  line L39 (-70.547, 41.635) -> (-70.547, 35.535)
  line L40 (-70.547, 35.535) -> (-74.177, 35.535)
  line L41 (-74.177, 35.535) -> (-74.177, 41.635)
  line L42 (-74.177, 41.635) -> (-70.547, 41.635)
  line L43 (-57.2555, 38.657) -> (-57.2555, 38.543)
  arc A0 (-61.0787, 42.085) -> (-57.2555, 38.543) centre (-60.755, 38.6) ccw
  line L44 (-61.0787, 42.085) -> (-60.4313, 42.085)
  arc A1 (-57.2555, 38.657) -> (-60.4313, 42.085) centre (-60.755, 38.6) ccw
  line L45 (-50.6145, 41.635) -> (-46.9845, 41.635)
  line L46 (-46.9845, 41.635) -> (-46.9845, 35.535)
  line L47 (-46.9845, 35.535) -> (-50.6145, 35.535)
  line L48 (-50.6145, 35.535) -> (-50.6145, 41.635)
  circle A2 centre (-80.08, 97.0008) radius 1.5
  circle A3 centre (-2.9851, 97) radius 1.5
  circle A4 centre (-80.08, 21.85) radius 1.5
  circle A5 centre (-2.9679, 21.85) radius 1.5
  circle A6 centre (-60.755, 38.6) radius 3.5
  dimension "d126" = 7
  constraint concentric A0 A6
  measures "d126" diameter of A6
sketch "Sketch12" plane through (0, 0, 0) normal (0, -1, 0) x (1, 0, 0)
  circle A0 centre (45.9348, 29.975) radius 3.5
  circle A1 centre (75.1296, 88.925) radius 3.5
  line L0 (52.98, 83.865) -> (71.9, 83.865)
  line L1 (71.9, 83.865) -> (71.9, 56.225)
  line L2 (71.9, 56.225) -> (52.98, 56.225)
  line L3 (52.98, 56.225) -> (52.98, 83.865)
  line L4 (38.05, 56.9) -> (38.05, 42.9)
  line L5 (38.05, 42.9) -> (24.05, 42.9)
  line L6 (24.05, 42.9) -> (24.05, 56.9)
  line L7 (24.05, 56.9) -> (38.05, 56.9)
  line L8 (19, 37.85) -> (19, 23.85)
  line L9 (19, 23.85) -> (5, 23.85)
  line L10 (5, 23.85) -> (5, 37.85)
  line L11 (5, 37.85) -> (19, 37.85)
  line L12 (5, 56.9) -> (19, 56.9)
  line L13 (19, 56.9) -> (19, 42.9)
  line L14 (19, 42.9) -> (5, 42.9)
  line L15 (5, 42.9) -> (5, 56.9)
  line L16 (24.05, 75.95) -> (38.05, 75.95)
  line L17 (38.05, 75.95) -> (38.05, 61.95)
  line L18 (38.05, 61.95) -> (24.05, 61.95)
  line L19 (24.05, 61.95) -> (24.05, 75.95)
  line L20 (5, 95) -> (19, 95)
  line L21 (19, 95) -> (19, 81)
  line L22 (19, 81) -> (5, 81)
  line L23 (5, 81) -> (5, 95)
  line L24 (38.05, 37.85) -> (38.05, 23.85)
  line L25 (38.05, 23.85) -> (24.05, 23.85)
  line L26 (24.05, 23.85) -> (24.05, 37.85)
  line L27 (24.05, 37.85) -> (38.05, 37.85)
  line L28 (19, 75.95) -> (19, 61.95)
  line L29 (19, 61.95) -> (5, 61.95)
  line L30 (5, 61.95) -> (5, 75.95)
  line L31 (5, 75.95) -> (19, 75.95)
  line L32 (24.05, 95) -> (38.05, 95)
  line L33 (38.05, 95) -> (38.05, 81)
  line L34 (38.05, 81) -> (24.05, 81)
  line L35 (24.05, 81) -> (24.05, 95)
  line L36 (83.08, 100) -> (0, 100)
  line L37 (0, 100) -> (0, 18.85)
  line L38 (0, 18.85) -> (83.08, 18.85)
  line L39 (83.08, 18.85) -> (83.08, 100)
  line L40 (70.547, 35.535) -> (70.547, 41.635)
  line L41 (70.547, 41.635) -> (74.177, 41.635)
  line L42 (74.177, 41.635) -> (74.177, 35.535)
  line L43 (74.177, 35.535) -> (70.547, 35.535)
  line L44 (57.2555, 38.543) -> (57.2555, 38.657)
  arc A2 (60.4313, 42.085) -> (57.2555, 38.657) centre (60.755, 38.6) ccw
  line L45 (60.4313, 42.085) -> (61.0787, 42.085)
  arc A3 (57.2555, 38.543) -> (61.0787, 42.085) centre (60.755, 38.6) ccw
  line L46 (46.9845, 41.635) -> (50.6145, 41.635)
  line L47 (50.6145, 41.635) -> (50.6145, 35.535)
  line L48 (50.6145, 35.535) -> (46.9845, 35.535)
  line L49 (46.9845, 35.535) -> (46.9845, 41.635)
  circle A4 centre (80.08, 97.0008) radius 1.5
  circle A5 centre (2.9851, 97) radius 1.5
  circle A6 centre (80.08, 21.85) radius 1.5
  circle A7 centre (2.9679, 21.85) radius 1.5
  circle A8 centre (45.8848, 89.005) radius 3.5
  circle A9 centre (74.9435, 29.945) radius 3.5
  line L50 (66.755, 44.6) -> (54.755, 44.6)
  line L51 (54.755, 44.6) -> (54.755, 32.6)
  line L52 (54.755, 32.6) -> (66.755, 32.6)
  line L53 (66.755, 32.6) -> (66.755, 44.6)
  line L54 (66.755, 44.6) -> (54.755, 32.6) construction
  line L55 (54.755, 44.6) -> (66.755, 32.6) construction
  point P0 (60.755, 38.6)
  dimension "d127" = 12
  dimension "d128" = 12
  constraint horizontal L50
  constraint perpendicular L50 L51
  constraint parallel L50 L52
  constraint parallel L51 L53
  constraint coincident L54 P0
  constraint coincident L55 P0
  constraint coincident P0 A2.centre
  measures "d127" distance of L51.end L52.end
  measures "d128" distance of L50.end L51.end
extrude "Extrude14" cut sketch "Sketch12" against normal blind 2.5 contours L50 L51 L52 L53
extrude "Extrude15" cut 1 faces at (52.98, 2, 74.6517) along direction (-1, 0, 0) blind 5
extrude "Extrude16" add 1 faces at (71.9, 1, 74.6517) along direction (-1, 0, 0) blind 5
sketch "Sketch13" plane through (0, -2, 0) normal (0, -1, 0) x (1, 0, 0)
  circle A0 centre (45.9348, 29.975) radius 1.85
  circle A1 centre (45.9348, 29.975) radius 2.5
  circle A2 centre (45.9348, 29.975) radius 2
  circle A3 centre (74.9, 29.9) radius 2
  circle A4 centre (75.1, 88.9) radius 2
  circle A5 centre (45.8889, 88.9935) radius 2
  dimension "d135" = 4
  dimension "d136" = 4
  dimension "d137" = 4
  dimension "d138" = 4
  constraint concentric A0 A2
  measures "d135" diameter of A2
  measures "d136" diameter of A3
  measures "d137" diameter of A4
  measures "d138" diameter of A5
extrude "Extrude17" cut sketch "Sketch13" against normal blind 4 contours A2 | A3 | A4 | A5
extrude "Extrude18" add sketch "Sketch11" against normal blind 3 contours L39 L40 L41 L42 | L45 L46 L47 L48
sketch "Sketch14" plane through (0, 3, 0) normal (0, 1, 0) x (-1, 0, 0)
  circle A0 centre (-2.9679, 21.85) radius 1.5
  circle A1 centre (-80.08, 21.85) radius 1.5
  circle A2 centre (-2.9851, 97) radius 1.5
  circle A3 centre (-80.08, 97.0008) radius 1.5
  line L0 (-57.2555, 38.657) -> (-57.2555, 38.543)
  arc A4 (-61.0787, 42.085) -> (-57.2555, 38.543) centre (-60.755, 38.6) ccw
  line L1 (-61.0787, 42.085) -> (-60.4313, 42.085)
  arc A5 (-57.2555, 38.657) -> (-60.4313, 42.085) centre (-60.755, 38.6) ccw
  line L2 (-38.05, 95) -> (-24.05, 95)
  line L3 (-24.05, 95) -> (-24.05, 81)
  line L4 (-24.05, 81) -> (-38.05, 81)
  line L5 (-38.05, 81) -> (-38.05, 95)
  line L6 (-19, 61.95) -> (-19, 75.95)
  line L7 (-19, 75.95) -> (-5, 75.95)
  line L8 (-5, 75.95) -> (-5, 61.95)
  line L9 (-5, 61.95) -> (-19, 61.95)
  line L10 (-38.05, 23.85) -> (-38.05, 37.85)
  line L11 (-38.05, 37.85) -> (-24.05, 37.85)
  line L12 (-24.05, 37.85) -> (-24.05, 23.85)
  line L13 (-24.05, 23.85) -> (-38.05, 23.85)
  line L14 (-19, 95) -> (-5, 95)
  line L15 (-5, 95) -> (-5, 81)
  line L16 (-5, 81) -> (-19, 81)
  line L17 (-19, 81) -> (-19, 95)
  line L18 (-38.05, 75.95) -> (-24.05, 75.95)
  line L19 (-24.05, 75.95) -> (-24.05, 61.95)
  line L20 (-24.05, 61.95) -> (-38.05, 61.95)
  line L21 (-38.05, 61.95) -> (-38.05, 75.95)
  line L22 (-19, 56.9) -> (-5, 56.9)
  line L23 (-5, 56.9) -> (-5, 42.9)
  line L24 (-5, 42.9) -> (-19, 42.9)
  line L25 (-19, 42.9) -> (-19, 56.9)
  line L26 (-19, 23.85) -> (-19, 37.85)
  line L27 (-19, 37.85) -> (-5, 37.85)
  line L28 (-5, 37.85) -> (-5, 23.85)
  line L29 (-5, 23.85) -> (-19, 23.85)
  line L30 (-38.05, 42.9) -> (-38.05, 56.9)
  line L31 (-38.05, 56.9) -> (-24.05, 56.9)
  line L32 (-24.05, 56.9) -> (-24.05, 42.9)
  line L33 (-24.05, 42.9) -> (-38.05, 42.9)
  line L34 (-83.08, 18.85) -> (0, 18.85)
  line L35 (0, 18.85) -> (0, 100)
  line L36 (0, 100) -> (-83.08, 100)
  line L37 (-83.08, 100) -> (-83.08, 18.85)
  line L38 (-66.9, 83.865) -> (-47.98, 83.865)
  line L39 (-47.98, 83.865) -> (-47.98, 56.225)
  line L40 (-47.98, 56.225) -> (-66.9, 56.225)
  line L41 (-66.9, 56.225) -> (-66.9, 83.865)
  circle A6 centre (-60.755, 38.6) radius 4.5
  dimension "d143" = 9
  constraint concentric A4 A6
  measures "d143" diameter of A6
extrude "Extrude19" cut sketch "Sketch14" against normal blind 0.5 contours A6
extrude "Extrude20" add 1 faces at (47.98, 2, 74.6517) along direction (1, 0, 0) blind 1.5
extrude "Extrude21" cut 1 faces at (49.48, 2, 74.6517) along direction (-1, 0, 0) blind 0.5
delete_face "DeleteFace1" 1 faces at (48.6368, -0.0011, 86.9204)
delete_face "DeleteFace2" 1 faces at (72.7162, -0.001, 86.4507)
delete_face "DeleteFace3" 1 faces at (72.5301, -0.001, 27.4707)
delete_face "DeleteFace4" 1 faces at (48.8841, -0.001, 28.1727)
extrude "Extrude22" add 4 faces at (44.9701, -2, 27.857) (77.0768, -2, 30.8265) (76.1742, -2, 90.9914) (44.34, -2, 90.7407) along direction (0, -1, 0) blind 2
fillet "Fillet2" radius 2 4 edges at (43.6039, 0, 30.879) (72.6127, 0, 30.849) (72.7988, 0, 89.829) (43.5539, 0, 89.909)
extrude "Extrude23" cut 1 faces at (60.9267, 2, 83.865) along direction (0, 0, 1) blind 2
extrude "Extrude24" cut 1 faces at (49.0231, 0, 85.8225) along direction (0, -1, 0) blind 0.7
extrude "Extrude25" add 1 faces at (60.6429, 2.5, 44.0958) along direction (0, -1, 0) blind 0.1